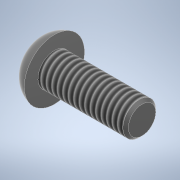
# Autodesk Inventor part: M3 X 8mm BHCS
Saved by Autodesk Inventor 2022 (Build 260153000, 153)
## iProperties
Created: 2022-05-12
Part Number: M3 X 8mm BHCS
Material: Generic
Document SubType Name: Modeling
Designer: Nick
Density: 1 g/cm^3
Appearance: Smooth - Black
Author: Nick
Autodesk Inventor part; units mm, degrees
ref_plane "YZ Plane" through (0, 0, 0) normal (1, 0, 0) x (0, 1, 0)
ref_plane "XZ Plane" through (0, 0, 0) normal (0, 1, 0) x (-1, 0, 0)
ref_plane "XY Plane" through (0, 0, 0) normal (0, 0, 1) x (1, 0, 0)
sketch "Sketch1" plane through (0, 0, 0) normal (0, 0, 1) x (1, 0, 0)
  line L0 (0, 0) -> (9.5, 0)
  line L1 (0, 0) -> (0, 1.5)
  arc A0 (1.5, 2.75) -> (0, 1.5) centre (1.8675, 0.784) ccw
  line L2 (1.5, 2.75) -> (1.5, 1.5)
  line L3 (1.5, 1.5) -> (9.5, 1.5)
  line L4 (9.5, 1.5) -> (9.5, 0)
  dimension "d0" = 1.5
  dimension "d1" = 3
  dimension "d2" = 5.5
  dimension "d3" = 3
  dimension "d4" = 8
  dimension "d5" = 2
  constraints: 10 end point, 3 vertical, 2 point on circle, 1 centre point, 1 horizontal, 1 perpendicular
  measures "d0" distance between parallel lines of L1 L2
  measures "d1" diameter of L3 L0
  measures "d2" diameter of L2.start L0
  measures "d3" diameter of L1.end L0
  measures "d4" distance of L2.end L3.end
  measures "d5" radius of A0
revolve "Revolution1" add sketch "Sketch1" angle 360 about axis through (0, 0, 0) along (1, 0, 0)
sketch "Sketch2" plane through (0, 0, 0) normal (-1, 0, 0) x (0, 0, 1)
  line L0 (0.5774, 1) -> (1.1547, 0)
  line L1 (1.1547, 0) -> (0.5774, -1)
  line L2 (0.5774, -1) -> (-0.5774, -1)
  line L3 (-0.5774, -1) -> (-1.1547, 0)
  line L4 (-1.1547, 0) -> (-0.5774, 1)
  line L5 (-0.5774, 1) -> (0.5774, 1)
  point P0 (0, 0)
  point P1 (0, 0)
  dimension "d7" = 2
  constraints: 12 end point, 1 coincident, 1 horizontal, 13 other
  measures "d7" distance between parallel lines of L2 L5
extrude "Extrusion1" cut sketch "Sketch2" against normal blind 1
thread "Thread1" size "M3x0.5" class "6g" standard "ANSI Metric M Profile" full length
chamfer "Chamfer1" distance 0.25 angle 45 1 edges at (9.5, -1.5, 0)
body "Solid1"
